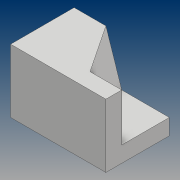
# Autodesk Inventor part: 49 (73500.000 mm^3)
Saved by Autodesk Inventor 2018 (Build 220112000, 112)
## iProperties
Created: 2020-09-18
Part Number: 49 (73500.000 mm^3)
Material: 一般
Document SubType Name: Modeling
Designer: 88697
Density: 1 g/cm^3
Appearance: 預設
Author: 88697
Autodesk Inventor part; units mm, degrees
ref_plane "YZ Plane" through (0, 0, 0) normal (1, 0, 0) x (0, 1, 0)
ref_plane "XZ Plane" through (0, 0, 0) normal (0, 1, 0) x (-1, 0, 0)
sketch "草圖1" plane through (0, 0, 0) normal (0, 1, 0) x (-1, 0, 0)
  line L0 (0, 0) -> (-60, 0)
  line L1 (-60, 0) -> (-60, -40)
  line L2 (-60, -40) -> (0, -40)
  line L3 (0, -40) -> (0, 0)
  dimension "d0" = 60
  dimension "d1" = 40
  constraints: 8 end point, 2 parallel, 1 horizontal, 1 perpendicular
  measures "d0" distance of L0.start L0.end
  measures "d1" distance of L2.end L0.start
extrude "擠出1" add sketch "草圖1" along normal blind 40
sketch "草圖2" plane through (60, 0, 0) normal (1, 0, 0) x (0, 0, -1)
  line L0 (0, 40) -> (30, 40)
  line L1 (30, 40) -> (30, 10)
  line L2 (30, 10) -> (0, 10)
  line L3 (0, 10) -> (0, 40)
  line L4 (40, 0) -> (40, 40) projected
  line L5 (0, 0) -> (40, 0) projected
  dimension "d4" = 10
  dimension "d5" = 10
  constraints: 8 end point, 2 parallel, 1 horizontal, 1 perpendicular
  measures "d4" distance between parallel lines of L4 L1
  measures "d5" distance between parallel lines of L5 L2
extrude "擠出2" cut sketch "草圖2" against normal blind 10
sketch "草圖6" plane through (0, 40, 0) normal (0, 1, 0) x (1, 0, 0)
  line L0 (0, 0) -> (60, 0) projected
  line L1 (60, 30) -> (60, 0) projected
  line L2 (0, 40) -> (0, 0) projected
  line L3 (50, 30) -> (60, 30) projected
  point P0 (20, 0)
  point P1 (30, 30)
  dimension "d12" = 30
  dimension "d13" = 20
  dimension "d14" = 0
  constraints: 1 point on line
  measures "d12" distance from line of L1 point (30, 30)
  measures "d13" distance from line of L2 point (20, 0)
  measures "d14" distance from line of L3 point (30, 30)
sketch "草圖7" plane through (0, 0, 0) normal (0, 0, 1) x (1, 0, 0)
  line L0 (60, 0) -> (60, 10) projected
  line L1 (60, 10) -> (50, 10) projected
  point P0 (0, 0)
  point P1 (40, 10)
  dimension "d15" = 20
  dimension "d16" = 0
  measures "d15" distance from line of L0 point (40, 10)
  measures "d16" distance from line of point (40, 10) L1
ref_plane "工作平面2" through (20, 40, 0) normal (-0.8017837, -0.5345225, -0.2672612) x (0.3162278, 0, -0.9486833)
sketch "草圖8" plane through (20, 40, 0) normal (-0.8017837, -0.5345225, -0.2672612) x (0.3162278, 0, -0.9486833)
  line L0 (-6.3246, -10.1419) -> (9.4868, 15.2128) projected
  line L1 (-1.8957, -3.0399) -> (37.7838, -3.0399)
  line L2 (37.7838, -3.0399) -> (37.7838, 41.2626)
  line L3 (37.7838, 41.2626) -> (-1.8957, 41.2626)
  line L4 (-1.8957, 41.2626) -> (-1.8957, -3.0399)
  point P0 (-6.3246, 23.6643)
  constraints: 8 end point, 2 parallel, 1 horizontal, 1 perpendicular, 1 point on line
extrude "擠出3" cut sketch "草圖8" against normal blind 50
sketch "草圖9" plane through (0, 40, 0) normal (0, 1, 0) x (1, 0, 0)
  line L0 (60, 30) -> (50, 30) projected
  line L1 (60, 40) -> (0, 40) projected
  line L2 (60, 30) -> (0, 30)
  line L3 (0, 30) -> (0, 40)
  line L4 (0, 40) -> (60, 40)
  line L5 (60, 40) -> (60, 30)
  point P0 (0, 0)
  constraints: 8 end point, 2 parallel, 1 horizontal, 1 perpendicular
extrude "擠出4" add sketch "草圖9" against normal up to next
sketch "草圖10" plane through (60, 0, -40) normal (1, 0, 0) x (0, 0, -1)
  line L0 (-10, 40) -> (0, 40) projected
  line L1 (0, 40) -> (-10, 40)
  line L2 (-10, 40) -> (-10, 0)
  line L3 (-10, 0) -> (0, 0)
  line L4 (0, 0) -> (0, 40)
  line L5 (-40, 0) -> (-40, 40) projected
  line L6 (0, 0) -> (-40, 0)
  line L7 (-40, 0) -> (-40, 10)
  line L8 (-40, 10) -> (0, 10)
  line L9 (0, 10) -> (0, 0)
  dimension "d21" = 0
  dimension "d22" = 10
  dimension "d23" = 10
  constraints: 16 end point, 4 parallel, 2 horizontal, 2 perpendicular, 2 point on line
  measures "d21" distance between parallel lines of L6 L3
  measures "d22" distance between parallel lines of L6 L8
  measures "d23" distance between parallel lines of L4 L2
extrude "擠出5" add sketch "草圖10" against normal up to next
delete faces "刪除面1" heal yes whole lump no faces at (50, 30, -29.8851) (49.8276, 20.2573, -29.8851)
